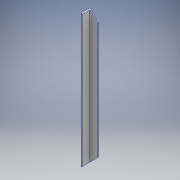
# Autodesk Inventor part: Profilé superieur cote
Saved by Autodesk Inventor 2017 (Build 210142000, 142)
## iProperties
Part Number: Profilé superieur cote
Project: 1400-PopCorn Machine
Material: Aluminium 6061
Catalog Web Link: http://www.frenchmakers.com/
Document SubType Name: Modeling
Designer: FABLAB Frenchmakers
Density: 2.7 g/cm^3
Appearance: Aluminium - Plat
Stock Number: 1400-06-01
RuleStatus: InUse
Company: FABLAB Frenchmakers
Author: Adrien MARY
Autodesk Inventor part; units mm, degrees
ref_plane "YZ Plane" through (0, 0, 0) normal (1, 0, 0) x (0, 1, 0)
ref_plane "XZ Plane" through (0, 0, 0) normal (0, 1, 0) x (-1, 0, 0)
ref_plane "XY Plane" through (0, 0, 0) normal (0, 0, 1) x (1, 0, 0)
sketch "Esquisse1" plane through (0, 0, 0) normal (0, 0, 1) x (1, 0, 0)
  line L0 (0, 0) -> (18.3, 0)
  line L1 (18.3, 0) -> (18.3, 2.2)
  line L2 (18.3, 2.2) -> (-2.2, 2.2)
  line L3 (-2.2, 2.2) -> (-2.2, -18.3)
  line L4 (-2.2, -18.3) -> (0, -18.3)
  line L5 (0, -18.3) -> (0, 0)
  dimension "Epaisseur_cornière" = 2.2
  dimension "Largueur" = 20.5
  constraints: 12 end point, 7 perpendicular, 1 horizontal
  measures "Epaisseur_cornière" distance between parallel lines of L2 L0
  measures "Largueur" distance of L1.end L2.end
extrude "Embase" add sketch "Esquisse1" along normal mid plane 310.4
sketch "Esquisse2" plane through (0, 0, 0) normal (0, 1, 0) x (-1, 0, 0)
  line L0 (2.2, 155.2) -> (-18.3, 134.7)
  line L1 (-18.3, 134.7) -> (-18.3, 155.2)
  line L2 (-18.3, 155.2) -> (2.2, 155.2)
  line L3 (-18.3, 155.2) -> (2.2, 155.2) construction
  line L4 (2.2, -155.2) -> (2.2, 155.2) construction
  line L5 (-18.3, -155.2) -> (-18.3, 155.2) construction
  point P0 (0, 0)
  dimension "d4" = 45
  constraints: 6 end point, 2 collinear, 1 vertical
  measures "d4" angle of L1 L0
extrude "Découpe à 45" cut sketch "Esquisse2" along normal through all both and the other way through all
mirror "Symétrie découpe" about plane through (0, 0, 0) normal (0, 0, 1) of "Découpe à 45"
